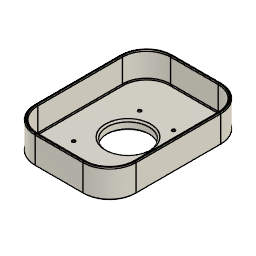
RV1-ELE-BKT-001_Lidar_Holder (Autodesk Fusion 360 design; units mm, degrees)
part number: 2026-02-18-13-50-08-782
Autodesk Fusion 360 part; units mm, degrees
sketch "Sketch1" plane through (0, 0, 0) normal (0, 0, 1) x (1, 0, 0)
  circle A0 centre (0, 0) radius 98.425
  circle A1 centre (0, 0) radius 101.6
  circle A2 centre (0, 0) radius 92.075
  line L0 (-54.5896, 85.6886) -> (54.5896, -85.6886)
  line L1 (71.842, -71.842) -> (-71.842, 71.842) construction
  line L2 (101.6, 0) -> (-101.6, 0) construction
  line L3 (0, -101.6) -> (0, 101.6)
  line L4 (54.5896, 85.6886) -> (-54.5896, -85.6886)
  line L5 (-71.842, -71.842) -> (71.8419, 71.8419) construction
  circle A3 centre (0, 0) radius 63.5
  spline S0 degree 5 poles (-53.9512, 165.1) (-57.8015, 164.6438) (-66.2924, 163.3711) (-79.1671, 160.3762) (-94.834, 153.7032) (-109.1061, 140.3344) (-117.2694, 122.5674) (-120.3596, 104.2145) (-120.6354, 92.1281) (-120.6083, 86.0123) (-120.6295, 83.4513) (-120.65, 82.55) knots 0.316926 0.316926 0.316926 0.316926 0.316926 0.316926 0.4 0.5 0.6 0.7 0.8 0.9 1 1 1 1 1 1
  line L6 (53.9512, 165.1) -> (-53.9512, 165.1)
  spline S1 degree 5 poles (120.65, 82.55) (120.6295, 83.4513) (120.6083, 86.0123) (120.6354, 92.1281) (120.3596, 104.2145) (117.2694, 122.5674) (109.1061, 140.3344) (94.834, 153.7032) (79.1671, 160.3762) (66.2924, 163.3711) (57.8015, 164.6438) (53.9512, 165.1) knots -1 -1 -1 -1 -1 -1 -0.9 -0.8 -0.7 -0.6 -0.5 -0.4 -0.316926 -0.316926 -0.316926 -0.316926 -0.316926 -0.316926
  line L7 (120.65, -82.55) -> (120.65, 82.55)
  line L8 (-120.65, 82.55) -> (-120.65, -82.55)
  spline S2 degree 5 poles (-120.65, -82.55) (-120.6295, -83.4513) (-120.6083, -86.0123) (-120.6354, -92.1281) (-120.3596, -104.2145) (-117.2694, -122.5674) (-109.1061, -140.3344) (-94.834, -153.7032) (-79.1671, -160.3762) (-66.2924, -163.3711) (-57.8015, -164.6438) (-53.9512, -165.1) knots -1 -1 -1 -1 -1 -1 -0.9 -0.8 -0.7 -0.6 -0.5 -0.4 -0.316926 -0.316926 -0.316926 -0.316926 -0.316926 -0.316926
  spline S3 degree 5 poles (53.9512, -165.1) (57.8015, -164.6438) (66.2924, -163.3711) (79.1671, -160.3762) (94.834, -153.7032) (109.1061, -140.3344) (117.2694, -122.5674) (120.3596, -104.2145) (120.6354, -92.1281) (120.6083, -86.0123) (120.6295, -83.4513) (120.65, -82.55) knots 0.316926 0.316926 0.316926 0.316926 0.316926 0.316926 0.4 0.5 0.6 0.7 0.8 0.9 1 1 1 1 1 1
  line L9 (-53.9512, -165.1) -> (53.9512, -165.1)
  dimension "d2" = 184.15
  dimension "d3" = 196.85
  dimension "d4" = 65
  dimension "d5" = 127
  constraint concentric A1 A3
  constraint coincident L3.start A1
  constraint coincident L3.end A1
  constraint vertical L3
  constraint coincident L2.start A1
  constraint coincident L2.end A1
  constraint perpendicular L2 L3
  constraint coincident L1.end A1
  constraint coincident L0.start A1
  constraint coincident L0.end A1
  constraint concentric A1 A2
  constraint concentric A0 A2
  constraint symmetric L0.start L4.start L3
  constraint symmetric L0.end L4.end L3
  measures "d2" diameter of A2
  measures "d3" diameter of A0
  measures "d4" angle of L0 L4
  measures "d5" diameter of A3
extrude "Locking Tabs" add sketch "Sketch1" along normal blind 4.75 contours A0 A2 L0 L3 | A0 A2 L0 L3 | A2 L0 L3 A3 | A2 L0 L3 A3 makes body 1 at (-39.9038, 76.8341, 4.75) makes body 2 at (7.6285, -86.2415, 0)
extrude "Locking Ring" add sketch "Sketch1" along normal blind 8.5 contours L0 L4 A3 | L3 L4 A3 | L0 L3 A3 | L0 L3 A3 | L0 L4 A3 | L3 L4 A3 bodies 1 2
move_body "Move1" bodies 1 to x (0.843391, -0.5373, 0) y (0.5373, 0.843391, 0) z (0, 0, 1) at (0, 0, 0)
extrude "Outer Lip" add sketch "Sketch1" along normal blind 7 from surface at 8.5 contours A0 A2 L0 L4 | A0 A1 L0 L4 | A0 A2 L3 L4 | A0 A1 L3 L4 | A0 A1 L0 L3 | A0 A2 L0 L3 | A0 A2 L0 L3 | A0 A1 L0 L3 | A2 L3 L4 A3 | A2 L0 L4 A3 | A0 A1 L3 L4 | A0 A2 L3 L4 | A2 L0 L3 A3 | A0 A2 L0 L4 | A0 A1 L0 L4 | A2 L0 L3 A3 | L0 L4 A3 | L3 L4 A3 | A2 L3 L4 A3 | L0 L3 A3 | A2 L0 L4 A3 | L0 L3 A3 | L0 L4 A3 | L3 L4 A3 bodies 1
scale "Scale1" factor 0.5 about (-101.6, 0, 15.5) bodies 1
move_body "Move2" bodies 1 to x (1, 0, 0) y (0, 1, 0) z (0, 0, 1) at (50.8, 0, 0)
sketch "Base Plate Sketch" plane through (0, 0, 15.5) normal (0, 0, 1) x (-1, 0, 0)
  circle A0 centre (0, 0) radius 50.8
  line L0 (-57.15, 164.908) -> (57.15, 164.908)
  line L1 (120.65, 101.408) -> (120.65, -101.408)
  line L2 (57.15, -164.908) -> (-57.15, -164.908)
  line L3 (-120.65, -101.408) -> (-120.65, 101.408)
  arc A1 (-57.15, 164.908) -> (-120.65, 101.408) centre (-57.15, 101.408) ccw
  arc A2 (57.15, -164.908) -> (120.65, -101.408) centre (57.15, -101.408) ccw
  arc A3 (-120.65, -101.408) -> (-57.15, -164.908) centre (-57.15, -101.408) ccw
  arc A4 (120.65, 101.408) -> (57.15, 164.908) centre (57.15, 101.408) ccw
  circle A5 centre (-20.25, -34.25) radius 1.55
  circle A6 centre (20.25, -34.25) radius 1.55
  circle A7 centre (28.25, 36.75) radius 1.55
  circle A8 centre (-28.25, 36.75) radius 1.55
  line L4 (28.25, 36.75) -> (-28.25, 36.75) construction
  line L5 (-28.25, 36.75) -> (0, 36.75) construction
  line L6 (20.25, -34.25) -> (-20.25, -34.25) construction
  line L7 (-20.25, -34.25) -> (0, -34.25) construction
  line L8 (-20.25, -34.25) -> (-28.25, -34.25) construction
  dimension "d15" = 63.5
  dimension "d16" = 63.5
  dimension "d24" = 40.5
  dimension "d25" = 3.1
  dimension "d26" = 3.1
  dimension "d27" = 3.1
  dimension "d28" = 3.1
  dimension "d57" = 56.5
  dimension "d58" = 8
  dimension "d59" = 71
  constraint horizontal L0
  constraint perpendicular L0 L1
  constraint parallel L0 L2
  constraint parallel L1 L3
  constraint coincident A0.centre origin
  constraint tangent L3 A1
  constraint tangent L0 A1
  constraint tangent L2 A2
  constraint tangent L1 A2
  constraint tangent L2 A3
  constraint tangent L3 A3
  constraint equal A2 A3
  constraint tangent L1 A4
  constraint tangent L0 A4
  constraint equal A2 A4
  constraint coincident A7.centre L4.start
  constraint coincident A8.centre L4.end
  constraint horizontal L4
  constraint midpoint L4 L5.end
  constraint coincident A6.centre L6.start
  constraint coincident A5.centre L6.end
  constraint horizontal L6
  constraint midpoint L6 L7.end
  constraint parallel L6 L8
  measures "d15" radius of A1
  measures "d16" radius of A2
  measures "d24" distance of A5.centre A6.centre
  measures "d25" diameter of A5
  measures "d26" diameter of A6
  measures "d27" diameter of A7
  measures "d28" diameter of A8
  measures "d57" distance of A7.centre A8.centre
  measures "d58" distance of A5.centre L8.end
  measures "d59" distance of A8.centre L8.end
extrude "Base Plate" add sketch "Base Plate Sketch" along normal blind 7 separate body contours A0 | L0 L1 L2 L3 A1 A2 A3 A4 | A5 | A6 | A7 | A8 makes body 3
scale "Scale2" factor 0.5 about (120.65, -101.408, 22.5) bodies 3
move_body "Move3" bodies 3 to x (1, 0, 0) y (0, 1, 0) z (0, 0, 1) at (-60.325, 50.7038, -3.5)
extrude "Base Plate Walls" add 1 faces at (20.1083, 16.9011, 19) along direction (0, 0, 1) blind 30 thin wall 3 inside on bodies 3 bodies 1 3
extrude "M2.5 Insert Holes" cut sketch "Base Plate Sketch" along normal blind 5 from surface at 2 contours A5 | A6 | A7 | A8 bodies 3 1
fillet "M2.5 Insert Chamfer" radius 0.3 4 edges at (21.6951, 33.6895, 19) (-18.8049, 33.6895, 19) (-26.8049, -37.3105, 19) (29.6951, -37.3105, 19) on bodies 3
sketch "Sketch3" plane through (0, 0, 7.75) normal (0, 0, -1) x (1, 0, 0)
  circle A0 centre (0, 0) radius 25
  line L0 (26.4419, -41.5054) -> (17.0593, -26.7777)
  arc A1 (17.0593, -26.7777) -> (0, 31.75) centre (0, 0) ccw
  line L1 (0, 31.75) -> (0, 49.2125)
  arc A2 (0, 49.2125) -> (-26.4419, 41.5054) centre (0, 0) ccw
  line L2 (-26.4419, 41.5054) -> (-17.0593, 26.7777)
  arc A3 (-17.0593, 26.7777) -> (0, -31.75) centre (0, 0) ccw
  line L3 (0, -31.75) -> (0, -49.2125)
  arc A4 (0, -49.2125) -> (26.4419, -41.5054) centre (0, 0) ccw
  dimension "d19" = 50
  measures "d19" diameter of A0
extrude "Wiring Hole" cut sketch "Sketch3" against normal blind 50.8 contours A0 bodies 1 3
combine "Combine1" operation add target body 3 tool bodies 1
fillet "Fillet3" radius 2 2 edges at (-23.3082, -9.0404, 7.75) (-23.3082, 9.0404, 19) on bodies 3
fillet "Locking Mech Chamfer" radius 1 33 edges at (-47.3622, 18.3701, 12) (51.0256, 73.1544, 49) (0, 82.4538, 49) (-51.0256, 73.1544, 49) (-60.325, -0.0002, 49) (-51.0256, -73.1548, 49) (0, -82.4542, 49) (51.0256, -73.1548, 49) (60.325, -0.0002, 49) (0, -79.4542, 49) (-48.9043, -71.0335, 49) (-57.325, -0.0002, 49) (-48.9043, 71.0331, 49) (0, 79.4538, 49) (48.9043, 71.0331, 49) (57.325, -0.0002, 49) (48.9043, -71.0335, 49) (-57.325, -0.0002, 19) (-48.9043, -71.0335, 19) (0, -79.4542, 19) (48.9043, -71.0335, 19) (57.325, -0.0002, 19) (48.9043, 71.0331, 19) (0, 79.4538, 19) (-48.9043, 71.0331, 19) (60.325, -0.0002, 15.5) (51.0256, -73.1548, 15.5) (0, -82.4542, 15.5) (-51.0256, -73.1548, 15.5) (-60.325, -0.0002, 15.5) (-51.0256, 73.1544, 15.5) (0, 82.4538, 15.5) (51.0256, 73.1544, 15.5) 13 faces at (12.2795, 33.4491, 7.75) (-25.7609, -1.2857, 8.1553) (-24.8758, -2.4892, 14.5833) (-25.7609, 1.2857, 18.5947) (-0.6726, -61.9443, 19) (29.975, -36.1221, 18.9997) (29.7065, -36.2199, 18.3) (-18.7935, 34.7801, 18.3) (-20.7472, 36.0171, 18.9997) (21.7065, 34.7801, 18.3) (19.7528, 36.0171, 18.9997) (-26.7935, -36.2199, 18.3) (-26.525, -36.1221, 18.9997) on bodies 3
